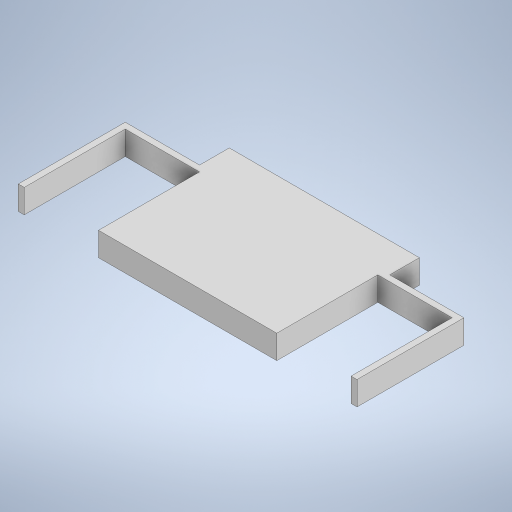
# Autodesk Inventor part: prent1
Saved by Autodesk Inventor 2023 (Build 270158000, 158)
## iProperties
Created: 2023-01-05
Part Number: prent1
Material: Ogólny
Document SubType Name: Modeling
Designer: User
Density: 1 g/cm^3
Appearance: Domyślna
Author: User
Autodesk Inventor part; units mm, degrees
ref_plane "YZ Plane" through (0, 0, 0) normal (1, 0, 0) x (0, 1, 0)
ref_plane "XZ Plane" through (0, 0, 0) normal (0, 1, 0) x (-1, 0, 0)
ref_plane "XY Plane" through (0, 0, 0) normal (0, 0, 1) x (1, 0, 0)
sketch "Szkic2" plane through (0, 0, 0) normal (0, 1, 0) x (-1, 0, 0)
  line L0 (14.0417, 4.5) -> (-14.4583, 4.5)
  line L1 (-14.4583, 4.5) -> (-14.4583, -4.5)
  line L2 (-14.4583, -4.5) -> (14.0417, -4.5)
  line L3 (14.0417, -4.5) -> (14.0417, 4.5)
  line L4 (20.5065, 0) -> (-20.5135, 0)
  line L5 (-0.0035, 27.5792) -> (-0.0035, -16.2627)
  line L6 (7.2917, -4.5) -> (-7.7083, -4.5)
  line L7 (-7.7083, -4.5) -> (-7.7083, -7)
  line L8 (-7.7083, -7) -> (7.2917, -7)
  line L9 (7.2917, -7) -> (7.2917, -4.5)
  line L10 (13.5417, 4.5) -> (13.5417, -4.5)
  line L11 (13.5417, -4) -> (7.2917, -4)
  line L12 (7.7917, -4.5) -> (7.7917, -7)
  line L13 (7.2917, -4) -> (7.2917, -4.5)
  line L14 (7.7917, -7) -> (7.2917, -7)
  line L15 (-8.2083, -4.5) -> (-8.2083, -7)
  line L16 (-8.2083, -7) -> (-7.7083, -7)
  line L17 (7.2917, -4) -> (7.2917, 4.5)
  line L18 (-7.7083, -4.5) -> (-7.7083, 4.5)
  line L19 (-13.9583, 4.5) -> (-13.9583, -4.5)
  line L20 (-7.7083, -4) -> (-13.9583, -4)
  line L21 (-7.7083, -4) -> (-7.7083, -4.5)
  point P0 (0, 0)
  dimension "d7" = 28.5
  dimension "d9" = 9
  dimension "d10" = 4.5
  dimension "d11" = 6.75
  dimension "d12" = 6.75
  dimension "d13" = 0.5
  dimension "d14" = 0.5
  dimension "d15" = 2.5
  dimension "d16" = 0.5
  dimension "d17" = 0.5
  dimension "d20" = 0.5
  dimension "d21" = 0.5
  constraints: 44 end point, 12 perpendicular, 12 point on line, 5 vertical, 4 horizontal, 4 parallel
  measures "d7" distance of L0.start L0.end
  measures "d9" distance of L2.end L0.start
  measures "d10" distance from line of L4 L0.start
  measures "d11" distance of L6.start L2.end
  measures "d12" distance of L1.end L6.end
  measures "d13" distance between parallel lines of L10 L3
  measures "d14" distance between parallel lines of L2 L11
  measures "d15" distance of L8.end L6.start
  measures "d16" distance of L12.end L8.end
  measures "d17" distance between parallel lines of L15 L7
  measures "d20" distance between parallel lines of L1 L19
  measures "d21" distance between parallel lines of L2 L20
extrude "Wyciągnięcie proste2" add sketch "Szkic2" along normal blind 2 contours L3 L4 L10 L0 | L3 L2 L10 L4 | L17 L4 L5 L0 | L5 L4 L18 L0 | L17 L13 L2 L5 L4 | L10 L2 L13 L11 | L5 L2 L18 L4 | L12 L14 L9 L2 | L19 L4 L1 L0 | L5 L8 L7 L2 | L2 L9 L8 L5 | L19 L2 L1 L4 | L18 L2 L19 L20 | L7 L16 L15 L2
